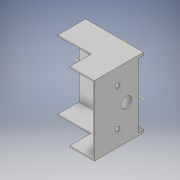
# Autodesk Inventor part: ProjectXBase
Saved by Autodesk Inventor 2019.4 (Build 234330000, 330)
## iProperties
Created: 2021-04-19
Part Number: ProjectXBase
Material: Generic
Document SubType Name: Modeling
Designer: ville
Density: 1 g/cm^3
Appearance: Default
Author: ville
Autodesk Inventor part; units mm, degrees
ref_plane "YZ Plane" through (0, 0, 0) normal (1, 0, 0) x (0, 1, 0)
ref_plane "XZ Plane" through (0, 0, 0) normal (0, 1, 0) x (-1, 0, 0)
ref_plane "XY Plane" through (0, 0, 0) normal (0, 0, 1) x (1, 0, 0)
sketch "Sketch1" plane through (0, 0, 0) normal (0, 0, 1) x (1, 0, 0)
  line L0 (-41.3322, 31.5) -> (12.6678, 31.5)
  line L1 (12.6678, 31.5) -> (12.6678, -31.5)
  line L2 (12.6678, -31.5) -> (-41.3322, -31.5)
  line L3 (-41.3322, -31.5) -> (-41.3322, 31.5)
  line L4 (-89.332, 0) -> (29.6678, 0) projected
  point P0 (0, 0)
  dimension "leveys" = 54
  dimension "pituus" = 63
  constraints: 8 end point, 2 parallel, 1 horizontal, 1 perpendicular, 1 other
  measures "leveys" distance between parallel lines of L3 L1
  measures "pituus" distance between parallel lines of L2 L0
extrude "Extrusion1" add sketch "Sketch1" along normal blind 1
sketch "Sketch2" plane through (0, 0, 1) normal (0, 0, 1) x (1, 0, 0)
  line L0 (12.6678, 31.5) -> (-41.3322, 31.5) projected
  line L1 (-41.3322, -31.5) -> (12.6678, -31.5) projected
  line L2 (12.6678, 31.5) -> (11.6678, 31.5)
  line L3 (11.6678, 31.5) -> (11.6678, -31.5)
  line L4 (11.6678, -31.5) -> (12.6678, -31.5)
  line L5 (12.6678, -31.5) -> (12.6678, 31.5)
  line L6 (11.6678, 30.5) -> (-41.3322, 30.5)
  line L7 (-41.3322, 31.5) -> (-41.3322, -31.5) projected
  line L8 (-41.3322, -30.5) -> (11.6678, -30.5)
  point P0 (0, 0)
  dimension "d4" = 1
  dimension "laita" = 1
  dimension "d9" = 1
  constraints: 12 end point, 4 point on line, 2 horizontal, 2 parallel, 2 perpendicular
  measures "d4" distance between parallel lines of L5 L3
  measures "laita" distance between parallel lines of L0 L6
  measures "d9" distance between parallel lines of L1 L8
extrude "Extrusion2" add sketch "Sketch2" along normal blind 40 contours L5 L1 L3 L0
sketch "Sketch3" plane through (12.6678, -31.5, 0) normal (1, 0, 0) x (0, 0, -1)
  circle A0 centre (-10.9634, 31.5) radius 5
  line L0 (-41, 0) -> (-41, 63) projected
  line L1 (-41, 31.5) -> (34.5285, 31.5) construction
  line L2 (-1, 63) -> (-1, 0) projected
  circle A1 centre (-19.1022, 49) radius 2.1
  circle A2 centre (-19.1022, 14) radius 2.1
  point P0 (0, 31.5)
  dimension "d7" = 10
  dimension "PIKKU" = 4.2
  dimension "d13" = 4.2
  dimension "d14" = 19.3
  dimension "d16" = 35
  constraints: 3 centre point, 2 end point, 1 midpoint, 1 perpendicular, 1 point on line, 1 symmetric about line
  measures "d7" diameter of A0
  measures "PIKKU" diameter of A1
  measures "d13" diameter of A2
  measures "d14" distance of A0.centre A1.centre
  measures "d16" distance of A2.centre A1.centre
extrude "Extrusion3" cut sketch "Sketch3" against normal up to next
sketch "Sketch4" plane through (-41.3322, 31.5, 0) normal (0, 1, 0) x (1, 0, 0)
  line L0 (0, 0) -> (54, 0) projected
  line L1 (54, 0) -> (0, 0)
  line L2 (0, 0) -> (0, -21)
  line L3 (0, -21) -> (31, -21)
  line L4 (54, -22.5156) -> (54, 0)
  line L5 (54, 0) -> (54, -41) projected
  line L6 (54, -41) -> (31, -41)
  line L7 (31, -41) -> (31, -21)
  line L8 (54, -22.5156) -> (54, -41)
  point P0 (41.3322, 0)
  dimension "d24" = 20
  dimension "d25" = 23
  constraints: 14 end point, 3 parallel, 2 horizontal, 2 perpendicular
  measures "d24" distance between parallel lines of L3 L6
  measures "d25" distance between parallel lines of L7 L5
extrude "Extrusion4" add sketch "Sketch4" along normal blind 1
mirror "Mirror1" about plane through (0, 0, 0) normal (0, 1, 0) of "Extrusion4"
sketch "Sketch7" plane through (0, 0, 0) normal (0, 0, -1) x (-1, 0, 0)
  line L0 (-12.6678, 30) -> (41.3322, 30)
  line L1 (-12.6678, -30) -> (41.3322, -30)
  line L2 (89.332, 0) -> (-29.6678, 0) projected
  line L3 (41.3322, -32.5) -> (41.3322, 32.5) projected
  line L4 (-12.6678, 32.5) -> (-12.6678, -32.5) projected
  line L5 (-12.6678, -32.5) -> (41.3322, -32.5) projected
  line L6 (-12.6678, 32.5) -> (41.3322, 32.5) projected
  point P0 (0, 0)
  dimension "d30" = 60
  constraints: 4 end point, 4 point on line, 2 horizontal, 1 other
  measures "d30" distance between parallel lines of L0 L1
extrude "Extrusion7" add sketch "Sketch7" along normal blind 5 contours L4 L6 L3 L0 | L1 L3 L5 L4
equation "\"d4\" = laita"
equation "\"d9\" = laita"
equation "\"d13\" = PIKKU"
body "Solid1"
